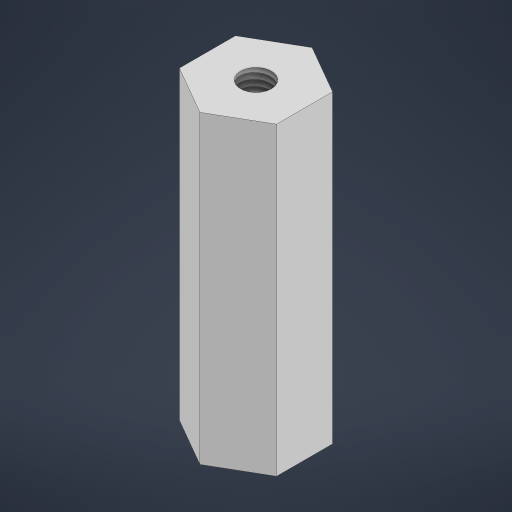
# Autodesk Inventor part: Gearbox4_003_Hexshaft
Saved by Autodesk Inventor 2024.4 (Build 284460000, 460)
## iProperties
Created: 2026-06-12
Part Number: Gearbox4_003_Hexshaft
Material: Generic
Document SubType Name: Modeling
Designer: stanr
Density: 1 g/cm^3
Appearance: Default
Author: stanr
Autodesk Inventor part; units mm, degrees
ref_plane "YZ Plane" through (0, 0, 0) normal (1, 0, 0) x (0, 1, 0)
ref_plane "XZ Plane" through (0, 0, 0) normal (0, 1, 0) x (-1, 0, 0)
ref_plane "XY Plane" through (0, 0, 0) normal (0, 0, 1) x (1, 0, 0)
sketch "Sketch1" plane through (0, 0, 0) normal (0, 1, 0) x (-1, 0, 0)
  line L0 (0, -7.3323) -> (-6.35, -3.6662)
  line L1 (-6.35, -3.6662) -> (-6.35, 3.6662)
  line L2 (-6.35, 3.6662) -> (0, 7.3323)
  line L3 (0, 7.3323) -> (6.35, 3.6662)
  line L4 (6.35, 3.6662) -> (6.35, -3.6662)
  line L5 (6.35, -3.6662) -> (0, -7.3323)
  circle A0 centre (0, 0) radius 2.0193
  point P0 (-3.175, 5.4993)
  point P1 (6.35, 0)
  dimension "d0" = 12.7
  dimension "d1" = 4.0386
  constraints: 12 end point, 2 coincident, 2 midpoint, 1 centre point, 1 vertical, 13 other
  measures "d0" distance from line of point (-3.175, 5.499) L5
  measures "d1" diameter of A0
extrude "Extrusion1" add sketch "Sketch1" along normal blind 39.878
thread "Thread1" size "10-32 UNF" class "2B" standard "ANSI Unified Screw Threads" full length
body "Solid1"
